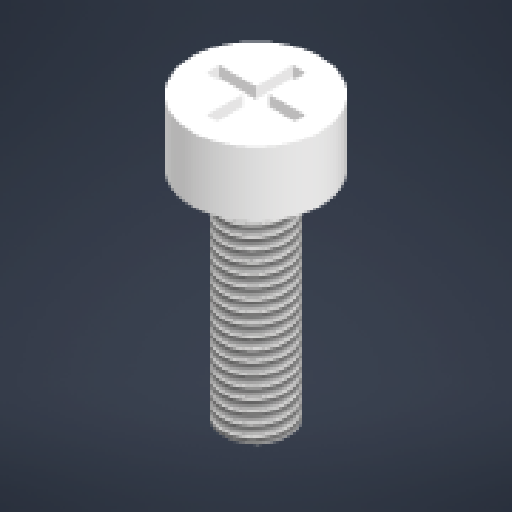
# Autodesk Inventor part: BoltM3-PI
Saved by Autodesk Inventor 2026.2 (Build 302298010, 298A)
## iProperties
Created: 2026-03-25
Part Number: BoltM3-PI
Material: PC/ABS Plastic
Document SubType Name: Modeling
Designer: usr
Density: 1.1 g/cm^3
Appearance: Smooth - White
Author: usr
Autodesk Inventor part; units mm, degrees
ref_plane "YZ Plane" through (0, 0, 0) normal (1, 0, 0) x (0, 1, 0)
ref_plane "XZ Plane" through (0, 0, 0) normal (0, 1, 0) x (-1, 0, 0)
ref_plane "XY Plane" through (0, 0, 0) normal (0, 0, 1) x (1, 0, 0)
sketch "Sketch1" plane through (0, 0, 0) normal (0, 1, 0) x (-1, 0, 0)
  circle A0 centre (0, 0) radius 1.5
  dimension "d0" = 3
  constraints: 1 centre point, 1 coincident
  measures "d0" diameter of A0
extrude "Extrusion1" add sketch "Sketch1" along normal blind 12
sketch "Sketch2" plane through (0, 12, 0) normal (0, 1, 0) x (1, 0, 0)
  circle A0 centre (0, 0) radius 3
  dimension "d3" = 6
  constraints: 1 centre point, 1 coincident
  measures "d3" diameter of A0
extrude "Extrusion2" add sketch "Sketch2" along normal blind 3
sketch "Sketch3" plane through (0, 15, 0) normal (0, 1, 0) x (1, 0, 0)
  line L0 (-2, -0.3) -> (-0.3, -0.3)
  line L1 (-0.3, -0.3) -> (-0.3, -2)
  line L2 (-0.3, -2) -> (0.3, -2)
  line L3 (0.3, -2) -> (0.3, -0.3)
  line L4 (0.3, -0.3) -> (2, -0.3)
  line L5 (2, -0.3) -> (2, 0.3)
  line L6 (2, 0.3) -> (0.3, 0.3)
  line L7 (0.3, 0.3) -> (0.3, 2)
  line L8 (0.3, 2) -> (-0.3, 2)
  line L9 (-0.3, 2) -> (-0.3, 0.3)
  line L10 (-2, 0.3) -> (-2, -0.3)
  line L11 (-2, 0.3) -> (-0.3, 0.3)
  circle A0 centre (0, 0) radius 3 projected
  point P0 (0, 0)
  dimension "d19" = 0.3
  dimension "d20" = 0.3
  dimension "d22" = 2
  dimension "d23" = 0
  dimension "d26" = 0.3
  dimension "d27" = 0.3
  constraints: 24 end point, 8 point on line, 7 perpendicular, 3 equal length, 1 horizontal
  measures "d19" distance from line of point (0, 0) L11
  measures "d20" distance from line of L7 point (0, 0)
  measures "d22" distance from line of L10 point (0, 0)
  measures "d23" distance of A0.centre point (0, 0)
  measures "d26" distance from line of L1 point (0, 0)
  measures "d27" distance from line of L4 A0.centre
extrude "Extrusion3" cut sketch "Sketch3" against normal blind 0.5 contours L10 L11 L9 L8 L7 L6 L5 L4 L3 L2 L1 L0
thread "Thread1" size "M3x0.5" class "6g" standard "ANSI Metric M Profile" full length
body "Solid1"
